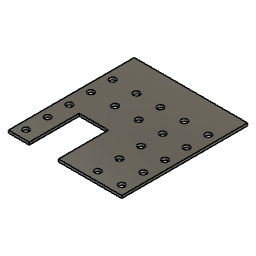
lid v3 (Autodesk Fusion 360 design; units mm, degrees)
Autodesk Fusion 360 part; units mm, degrees
sketch "Sketch1" plane through (0, 0, 0) normal (0, 0, 1) x (1, 0, 0)
  line L0 (0, 0) -> (272.2, 0)
  line L1 (272.2, 0) -> (272.2, 302.2)
  line L2 (272.2, 302.2) -> (0, 302.2)
  line L3 (0, 302.2) -> (0, 0)
  dimension "d1" = 272.2
  dimension "d2" = 302.2
  constraint horizontal L0
  constraint vertical L1
  constraint horizontal L2
  constraint vertical L3
  constraint coincident L0.start L3.end
  measures "d1" distance of L0.start L0.end
  measures "d2" distance of L0.start L2.end
extrude "Extrude1" add sketch "Sketch1" against normal blind 6
sketch "Sketch2" plane through (0, 0, 0) normal (0, 0, 1) x (-1, 0, 0)
  line L0 (0, -302.2) -> (0, 0)
  line L1 (0, 0) -> (-272.2, 0)
  line L2 (-272.2, 0) -> (-272.2, -302.2)
  line L3 (-272.2, -302.2) -> (0, -302.2)
  line L4 (-50, 0) -> (-120, 0)
  line L5 (-120, 0) -> (-120, -120)
  line L6 (-120, -120) -> (-50, -120)
  line L7 (-50, -120) -> (-50, 0)
  circle A0 centre (-20, -230.2) radius 7.5
  circle A1 centre (-77.5, -230.2) radius 7.5
  circle A2 centre (-135, -230.2) radius 7.5
  circle A3 centre (-192.5, -230.2) radius 7.5
  circle A4 centre (-250, -230.2) radius 7.5
  circle A5 centre (-20, -178.2) radius 7.5
  circle A6 centre (-77.5, -178.2) radius 7.5
  circle A7 centre (-135, -178.2) radius 7.5
  circle A8 centre (-192.5, -178.2) radius 7.5
  circle A9 centre (-250, -178.2) radius 7.5
  circle A10 centre (-20, -126.2) radius 7.5
  circle A11 centre (-192.5, -126.2) radius 7.5
  circle A12 centre (-250, -126.2) radius 7.5
  circle A13 centre (-20, -74.2) radius 7.5
  circle A14 centre (-192.5, -74.2) radius 7.5
  circle A15 centre (-250, -74.2) radius 7.5
  circle A16 centre (-20, -22.2) radius 7.5
  circle A17 centre (-192.5, -22.2) radius 7.5
  circle A18 centre (-250, -22.2) radius 7.5
  dimension "d5" = 70
  dimension "d6" = 120
  dimension "d7" = 50
  constraint horizontal L4
  constraint vertical L5
  constraint horizontal L6
  constraint vertical L7
  constraint coincident L1 L4.start
  measures "d5" distance of L4.start L4.end
  measures "d6" distance of L4.start L6.end
  measures "d7" distance of L0 L7
extrude "Extrude2" cut sketch "Sketch2" against normal up to surface (6 mm away) contours L1 L4 L5 L6 L7 | A0 | A1 | A2 | A3 | A4 | A5 | A6 | A7 | A8 | A9 | A10 | A11 | A12 | A13 | A14 | A15 | A16 | A17 | A18
